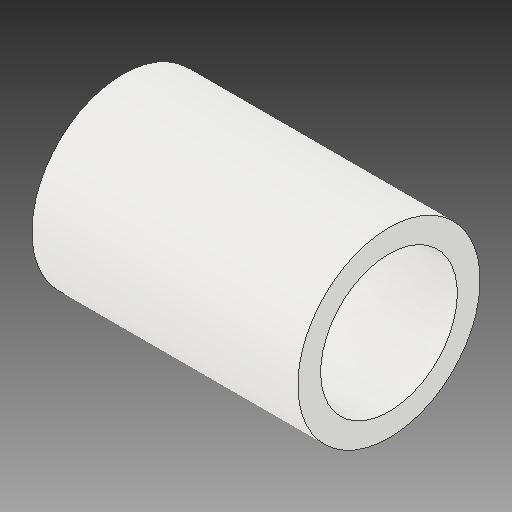
# Autodesk Inventor part: 363-52
Saved by Autodesk Inventor 2019 (Build 230136000, 136)
## iProperties
Company: Autodesk Inc.
Created: 2017-03-19
Part Number: 363-52
Material: Generic
Document SubType Name: Modeling
Designer: Autodesk Inc.
Density: 1 g/cm^3
Appearance: Default
Mass: 2.05406 g
Surface Area: 22.2999 cm^2
Volume: 2.05406 cm^3
Author: Inventor
Autodesk Inventor part; units mm, degrees
ref_plane "YZ Plane" through (0, 0, 0) normal (1, 0, 0) x (0, 1, 0)
ref_plane "XZ Plane" through (0, 0, 0) normal (0, 1, 0) x (-1, 0, 0)
ref_plane "XY Plane" through (0, 0, 0) normal (0, 0, 1) x (1, 0, 0)
sketch "Sketch1" plane through (0, 0, 0) normal (1, 0, 0) x (0, 1, 0)
  circle A0 centre (0, 0) radius 6
  circle A1 centre (0, 0) radius 8
  dimension "d1" = 16
  dimension "d2" = 12
  constraints: 2 centre point, 2 coincident
  measures "d1" diameter of A1
  measures "d2" diameter of A0
extrude "Extrusion1" add sketch "Sketch1" along normal blind 23.351
body "Solid1"
